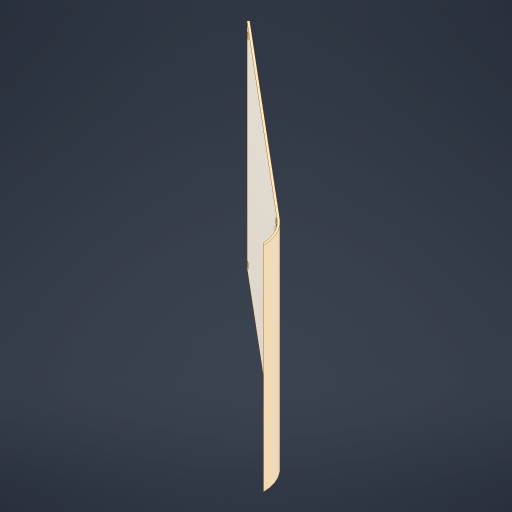
# Autodesk Inventor part: intakeabs
Saved by Autodesk Inventor 2023 (Build 270158000, 158)
## iProperties
Created: 2023-02-25
Part Number: intakeabs
Material: Polyethylene, High Density
Document SubType Name: Modeling
Designer: Windows Macbook
Density: 0.952 g/cm^3
Appearance: Smooth - Off-White
Author: Windows Macbook
Autodesk Inventor part; units mm, degrees
ref_plane "YZ Plane" through (0, 0, 0) normal (1, 0, 0) x (0, 1, 0)
ref_plane "XZ Plane" through (0, 0, 0) normal (0, 1, 0) x (-1, 0, 0)
ref_plane "XY Plane" through (0, 0, 0) normal (0, 0, 1) x (1, 0, 0)
sketch "Sketch1" plane through (0, 0, 0) normal (0, 1, 0) x (-1, 0, 0)
  line L0 (131.6241, -133.8819) -> (133.2116, -133.8819)
  arc A0 (0, 0) -> (11.8436, -25.4008) centre (33.1555, -0.0022) ccw
  line L1 (11.8436, -25.4008) -> (167.5038, -156.0152)
  arc A1 (1.5875, 0) -> (1.5875, -0.0044) centre (33.1555, -0.0022) ccw
  line L2 (12.864, -24.1847) -> (168.5242, -154.7991)
  line L3 (168.5242, -154.7991) -> (167.5038, -156.0152)
  line L4 (0, -0.0044) -> (1.6297, -1.6341)
  arc A2 (1.6297, -1.6341) -> (12.864, -24.1847) centre (33.1555, -0.0022) ccw
  dimension "d15" = 1.5875
  constraints: 10 end point, 7 point on circle, 3 centre point, 1 horizontal
  measures "d15" radial gap between concentric circles of A0 A1
extrude "Extrusion1" add sketch "Sketch1" along normal blind 177.8
sketch "Sketch2" plane through (-12.864, 0, -24.1847) normal (-0.6427876, 0, 0.7660444) x (0.7660444, 0, 0.6427876)
  line L0 (0, 0) -> (0, 177.8) projected
  line L1 (-203.2, 0) -> (-185.2395, 0) construction
  line L2 (0, 165.1) -> (17.9605, 165.1) construction
  line L3 (-203.2, 165.1) -> (-185.2395, 165.1) construction
  point P0 (25.4, 0)
  point P1 (-6.35, 6.35)
  point P2 (-196.85, 6.35)
  point P3 (-203.2, 177.8)
  point P4 (-6.35, 171.45)
  point P5 (-196.85, 171.45)
  constraints: 6 end point, 3 horizontal
hole "Hole1" at (-163.6598, 6.35, -150.7174) at (-163.6598, 171.45, -150.7174) at (-17.7284, 171.45, -28.2664) at (-17.7284, 6.35, -28.2664) direction (0.6427876, 0, -0.7660444) diameter 4.7625 end through all
body "Solid1"
